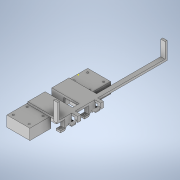
# Autodesk Inventor part: shell 6.0 screw
Saved by Autodesk Inventor 2020.2 (Build 242310000, 310)
## iProperties
Created: 2020-02-28
Part Number: shell 6.0 screw
Material: Generic
Document SubType Name: Modeling
Designer: ColinP
Density: 1 g/cm^3
Appearance: Default
Author: ColinP
Autodesk Inventor part; units mm, degrees
ref_plane "YZ Plane" through (0, 0, 0) normal (1, 0, 0) x (0, 1, 0)
ref_plane "XZ Plane" through (0, 0, 0) normal (0, 1, 0) x (-1, 0, 0)
ref_plane "XY Plane" through (0, 0, 0) normal (0, 0, 1) x (1, 0, 0)
sketch "Sketch1" plane through (0, 0, 0) normal (0, 1, 0) x (-1, 0, 0)
  line L0 (0, 0) -> (8, 0)
  line L1 (8, 0) -> (8, 98.298)
  line L2 (8, 98.298) -> (0, 98.298)
  line L3 (0, 98.298) -> (0, 0)
  line L4 (8, 0) -> (0, 0)
  line L5 (0, 0) -> (0, -4)
  line L6 (0, -4) -> (8, -4)
  line L7 (8, -4) -> (8, 0)
  line L8 (8, 98.298) -> (0, 98.298)
  line L9 (0, 98.298) -> (0, 102.298)
  line L10 (0, 102.298) -> (8, 102.298)
  line L11 (8, 102.298) -> (8, 98.298)
  dimension "d0" = 8
  dimension "d1" = 98.298
  dimension "d2" = 8
  dimension "d3" = 4
  dimension "d4" = 4
  constraints: 24 end point, 6 parallel, 3 horizontal, 3 perpendicular
  measures "d0" distance of L2.end L1.end
  measures "d1" distance of L1.end L0.end
  measures "d2" distance of L6.end L5.end
  measures "d3" distance of L5.end L4.end
  measures "d4" distance of L8.end L9.end
extrude "Extrusion1" add sketch "Sketch1" along normal blind 4 contours L3 L2 L1 L0
extrude "Extrusion2" add sketch "Sketch1" along normal blind 34 contours L0 L7 L6 L5
sketch "Sketch2" plane through (0, 0, 0) normal (0, -1, 0) x (1, 0, 0)
  line L0 (0, 0) -> (0, 19.558)
  line L1 (0, 98.298) -> (0, 0) projected
  line L2 (0, 19.558) -> (0, 35.6705)
  line L3 (0, 35.6705) -> (0, 48.3705)
  line L4 (0, 48.3705) -> (-8, 48.3705)
  line L5 (-8, 0) -> (-8, 98.298) projected
  line L6 (-8, 19.558) -> (-8, 48.3705)
  line L7 (0, 19.558) -> (-8, 19.558)
  dimension "d9" = 19.558
  dimension "d10" = 16.1125
  dimension "d11" = 12.7
  constraints: 12 end point, 5 point on line, 2 perpendicular, 1 collinear
  measures "d9" distance of L0.start L0.end
  measures "d10" distance of L0.end L2.end
  measures "d11" distance of L2.end L3.end
extrude "Extrusion3" add sketch "Sketch2" along normal blind 25
sketch "Sketch3" plane through (0, 0, -4) normal (1, 0, 0) x (0, 0, -1)
  line L0 (-52.3705, -25) -> (-23.558, -25)
  line L1 (-37.9642, -25) -> (-37.9642, -17.7991)
  line L2 (-37.9642, -17.7991) -> (-31.5508, -17.7991)
  line L3 (-31.5508, -17.7991) -> (-44.3778, -17.7991)
  line L4 (-44.3778, -17.7991) -> (-41.1646, -12.2338)
  line L5 (-44.3778, -17.7991) -> (-37.9516, -17.7991) construction
  line L6 (-41.1646, -12.2338) -> (-34.7385, -12.2338)
  line L7 (-34.7385, -12.2338) -> (-31.5253, -17.7991)
  line L8 (-31.5253, -17.7991) -> (-34.7385, -23.3644)
  line L9 (-34.7385, -23.3644) -> (-41.1647, -23.3644)
  line L10 (-41.1647, -23.3644) -> (-44.3778, -17.7991)
  line L11 (-23.558, 0) -> (-23.558, -25)
  line L12 (-52.3705, 0) -> (-52.3705, -25)
  line L13 (-23.558, -25) -> (-52.3705, -25)
  line L14 (-52.3705, -25) -> (-52.3705, -13.8875)
  line L15 (-23.558, -13.8875) -> (-23.558, -25)
  line L16 (-31.5253, -17.7991) -> (-23.558, -17.7991)
  line L17 (-44.3778, -17.7991) -> (-52.3705, -17.7991)
  point P0 (-4, 0)
  point P1 (-37.9642, -23.3644)
  dimension "d14" = 7.2009
  dimension "d15" = 6.4135
  dimension "d16" = 12.827
  dimension "d17" = 6.4262
  dimension "d18" = 60
  dimension "d19" = 6.4262
  dimension "d20" = 120
  dimension "d21" = 120
  dimension "d22" = 6.4262
  dimension "d23" = 120
  dimension "d24" = 6.4262
  dimension "d25" = 120
  constraints: 30 end point, 6 horizontal, 5 point on line, 3 parallel, 1 equal length, 1 midpoint, 1 perpendicular, 1 vertical
  measures "d14" distance of L1.start L1.end
  measures "d15" distance of L1.end L2.end
  measures "d16" distance of L2.end L3.end
  measures "d17" distance of L3.end L4.end
  measures "d18" angle of L5 L4
  measures "d19" distance of L4.end L6.end
  measures "d20" angle of L4 L6
  measures "d21" angle of L6 L7
  measures "d22" distance of L7.end L8.end
  measures "d23" angle of L7 L8
  measures "d24" distance of L8.end L9.end
  measures "d25" angle of L8 L9
extrude "Extrusion4" cut sketch "Sketch3" against normal blind 25.4
sketch "Sketch4" plane through (0, 0, -4) normal (1, 0, 0) x (0, 0, -1)
  line L0 (0, 0) -> (-23.558, 0) projected
  line L1 (-23.558, 0) -> (-29.558, 0)
  line L2 (-29.558, 0) -> (-29.558, -12.8016)
  line L3 (-29.558, -12.8016) -> (-23.558, -12.8016)
  line L4 (-23.558, -12.8016) -> (-23.558, 0)
  line L5 (-52.3705, 0) -> (-52.3705, -25) projected
  line L6 (-52.3705, 0) -> (-46.3761, 0)
  line L7 (-46.3761, 0) -> (-46.3761, -12.8016)
  line L8 (-46.3761, -12.8016) -> (-52.3705, -12.8016)
  line L9 (-52.3705, -12.8016) -> (-52.3705, 0)
  point P0 (-4, 0)
  point P1 (-52.3705, -13.8875)
  dimension "d28" = 6
  dimension "d29" = 12.8016
  dimension "d30" = 5.9944
  dimension "d31" = 12.8016
  constraints: 16 end point, 4 parallel, 2 horizontal, 2 perpendicular
  measures "d28" distance of L3.end L2.end
  measures "d29" distance of L2.end L1.end
  measures "d30" distance of L7.end L8.end
  measures "d31" distance of L6.end L7.end
extrude "Extrusion5" cut sketch "Sketch4" against normal blind 25.4
sketch "Sketch6" plane through (0, 0, -4) normal (1, 0, 0) x (0, 0, -1)
  line L0 (-29.558, -12.8016) -> (-29.558, 0) projected
  line L1 (-29.558, 0) -> (-31.558, 0)
  line L2 (-31.558, 0) -> (-31.558, -12.8016)
  line L3 (-31.558, -12.8016) -> (-29.558, -12.8016)
  line L4 (-29.558, -12.8016) -> (-29.558, 0)
  line L5 (-46.3761, -12.8016) -> (-46.3761, 0) projected
  line L6 (-46.3761, 0) -> (-44.3761, 0)
  line L7 (-44.3761, 0) -> (-44.3761, -12.8016)
  line L8 (-44.3761, -12.8016) -> (-46.3761, -12.8016)
  line L9 (-46.3761, -12.8016) -> (-46.3761, 0)
  point P0 (-4, 0)
  dimension "d44" = 2
  dimension "d45" = 12.8016
  dimension "d46" = 2
  constraints: 16 end point, 4 parallel, 2 horizontal, 2 perpendicular, 1 point on line
  measures "d44" distance of L3.end L2.end
  measures "d45" distance of L2.end L1.end
  measures "d46" distance of L7.end L8.end
extrude "Extrusion6" cut sketch "Sketch6" against normal blind 25.4
sketch "Sketch5" plane through (0, -17.7991, 19.558) normal (0, -1, 0) x (1, 0, 0)
  line L0 (-8, 0) -> (0, 0) projected
  line L1 (-4, 0) -> (-4, 28.8125)
  line L2 (-8, 28.8125) -> (0, 28.8125) projected
  line L3 (-4, 14.4063) -> (-4, 4.4063)
  line L4 (-4, 14.4063) -> (6, 14.4063) construction
  line L5 (-4, 4.4063) -> (-4, 24.4062)
  point P0 (0, -19.558)
  dimension "d34" = 10
  dimension "d35" = 90
  dimension "d36" = 20
  constraints: 8 end point, 3 midpoint, 1 horizontal, 1 perpendicular, 1 point on line, 1 vertical
  measures "d34" distance of L3.start L3.end
  measures "d35" angle of L3 L4
  measures "d36" distance of L3.end L5.end
hole "Hole1" at (-4, -17.7991, 23.9642) at (-4, -17.7991, 43.9642) direction (0, 1, 0) diameter 3.4 depth 4.9975 clearance for "Flat Head Machine Screw" size "M3" standard "Ansi Metric M Profile"
sketch "Sketch14" plane through (0, 4, 0) normal (0, 1, 0) x (1, 0, 0)
  line L0 (-8, -30.7385) -> (-8, -37.1647) projected
  line L1 (0, -30.7385) -> (-8, -30.7385) projected
  line L2 (0, -37.1647) -> (0, -30.7385) projected
  line L3 (0, -37.1647) -> (-8, -37.1647) projected
  line L4 (-8, -33.9515) -> (-8, -17.7115)
  line L5 (-8, -17.7115) -> (-59.53, -17.7116)
  line L6 (-59.53, -17.7116) -> (-59.53, -50.1916)
  line L7 (-59.53, -50.1916) -> (-8, -50.1915)
  line L8 (-8, -50.1915) -> (-8, -17.7115)
  point P0 (0, 0)
  point P1 (-8, -37.1647)
  point P2 (-8, -30.7385)
  dimension "d78" = 16.24
  dimension "d79" = 51.53
  dimension "d80" = 32.48
  dimension "d81" = 90
  dimension "d82" = 90
  constraints: 10 end point, 2 perpendicular, 1 midpoint
  measures "d78" distance of L4.start L4.end
  measures "d79" distance of L4.end L5.end
  measures "d80" distance of L5.end L6.end
  measures "d81" angle of L6 L5
  measures "d82" angle of L7 L6
extrude "Extrusion11" add sketch "Sketch14" against normal blind 4 contours L0 L8 L7 L6 L5 L4
sketch "Sketch15" plane through (0, 0, 0) normal (0, -1, 0) x (1, 0, 0)
  line L0 (-59.53, 19.7116) -> (-59.53, 17.7116)
  line L1 (-8, 17.7115) -> (-59.53, 17.7116) projected
  line L2 (-59.53, 17.7116) -> (-57.53, 17.7116)
  line L3 (-57.53, 17.7116) -> (-57.53, 19.7116)
  line L4 (-57.53, 19.7116) -> (-59.53, 19.7116)
  line L5 (-59.53, 19.7116) -> (-59.53, 17.7116)
  line L6 (-59.53, 50.1916) -> (-59.53, 17.7116) projected
  line L7 (-59.53, 50.1916) -> (-38.53, 50.1916)
  line L8 (-38.53, 50.1916) -> (-38.53, 48.1916)
  line L9 (-38.53, 48.1916) -> (-59.53, 48.1916)
  line L10 (-59.53, 48.1916) -> (-59.53, 50.1916)
  line L11 (-38.53, 48.1916) -> (-57.53, 48.1916)
  line L12 (-57.53, 48.1916) -> (-57.53, 19.7116)
  line L13 (-57.53, 19.7116) -> (-38.53, 19.7116)
  line L14 (-38.53, 19.7116) -> (-38.53, 48.1916)
  line L15 (-38.53, 19.7116) -> (-57.53, 19.7116)
  line L16 (-57.53, 19.7116) -> (-57.53, 17.7116)
  line L17 (-57.53, 17.7116) -> (-38.53, 17.7116)
  line L18 (-38.53, 17.7116) -> (-38.53, 19.7116)
  line L19 (-8, -4) -> (-8, 17.7115) projected
  line L20 (0, -4) -> (-8, -4) projected
  line L21 (0, 27.558) -> (0, -4) projected
  line L22 (0, 27.558) -> (-8, 27.558) projected
  line L23 (-8, 40.3761) -> (-8, 27.558) projected
  line L24 (0, 40.3761) -> (-8, 40.3761) projected
  line L25 (0, 98.298) -> (0, 40.3761) projected
  line L26 (-8, 50.1915) -> (-8, 98.298) projected
  line L27 (-8, 50.1915) -> (-59.53, 50.1916) projected
  line L28 (-59.53, 50.1916) -> (-59.53, 17.7116) projected
  line L29 (-59.53, 17.7116) -> (-8, 17.7115) projected
  line L30 (-8, 98.298) -> (0, 98.298) projected
  point P0 (0, 0)
  point P1 (-38.53, 17.7116)
  dimension "d87" = 2
  dimension "d88" = 2
  dimension "d89" = 21
  dimension "d90" = 2
  constraints: 34 end point, 8 parallel, 4 horizontal, 4 perpendicular
  measures "d87" distance of L4.end L3.end
  measures "d88" distance of L3.end L2.end
  measures "d89" distance of L8.end L9.end
  measures "d90" distance of L7.end L8.end
extrude "Extrusion12" add sketch "Sketch15" along normal blind 36 contours L4 L3 L1 L0 | L6 L9 L12 L4 | L13 L18 L1 L3 | L6 L7 L8 L9
sketch "Sketch16" plane through (-38.53, 0, 48.1916) normal (1, 0, 0) x (0, 0, -1)
  line L0 (7.8155, 0) -> (20.6335, 0) projected
  line L1 (14.2245, 0) -> (14.2245, -17.78)
  line L2 (14.2245, -17.78) -> (14.2245, -25.78)
  line L3 (14.2245, -25.78) -> (31.7245, -25.78)
  line L4 (31.7245, -25.78) -> (-3.2755, -25.78)
  line L5 (-3.2755, -25.78) -> (-3.2755, -22.28)
  line L6 (-3.2755, -22.28) -> (-2, -22.28)
  line L7 (-2, 0) -> (-2, -36) projected
  line L8 (-2, -22.28) -> (-7, -22.28)
  line L9 (-7, -22.28) -> (-7, -29.28)
  line L10 (-7, -22.28) -> (0, -22.28) construction
  line L11 (-7, -29.28) -> (-2, -29.28)
  line L12 (-2, -22.28) -> (-2, -29.28)
  line L13 (30.48, 0) -> (30.48, -36) projected
  line L14 (30.48, -29.28) -> (35.48, -29.28)
  line L15 (35.48, -29.28) -> (35.48, -22.28)
  line L16 (35.48, -22.28) -> (30.48, -22.28)
  circle A0 centre (-3.2755, -25.78) radius 1.7
  circle A1 centre (31.7245, -25.78) radius 1.7
  point P0 (48.1916, 0)
  point P1 (-2, -26.9039)
  point P2 (-3.2755, -24.08)
  point P3 (30.48, -24.6219)
  point P4 (30.48, -26.9381)
  point P5 (-2, -24.6561)
  point P6 (32.98, -22.28)
  point P7 (-3.5, -22.28)
  dimension "d93" = 17.78
  dimension "d94" = 8
  dimension "d95" = 180
  dimension "d96" = 17.5
  dimension "d97" = 90
  dimension "d98" = 35
  dimension "d99" = 3.5
  dimension "d100" = 5
  dimension "d101" = 7
  dimension "d102" = 90
  dimension "d103" = 5
  dimension "d104" = 3.4
  dimension "d105" = 3.4
  constraints: 28 end point, 8 perpendicular, 8 point on line, 3 midpoint, 2 centre point, 2 coincident, 2 vertical, 1 collinear, 1 horizontal, 1 horizontal alignment
  measures "d93" distance of L1.start L1.end
  measures "d94" distance of L1.end L2.end
  measures "d95" angle of L2 L1
  measures "d96" distance of L2.end L3.end
  measures "d97" angle of L3 L2
  measures "d98" distance of L3.end L4.end
  measures "d99" distance of L4.end L5.end
  measures "d100" distance of L6.end L8.end
  measures "d101" distance of L8.end L9.end
  measures "d102" angle of L9 L10
  measures "d103" distance of L14.start L14.end
  measures "d104" diameter of A0
  measures "d105" diameter of A1
extrude "Extrusion13" cut sketch "Sketch16" against normal blind 25.4 contours A1 L13 L3 | L3 L13 A1 | L13 A1 | A0 L7 L4 | L4 L7 A0 | L7 A0 L5 L4 | L4 L5 A0 L7
extrude "Extrusion14" add sketch "Sketch16" against normal blind 6.4262 contours L13 L16 L15 L14 A1 | A0 L5 L6 L7 | L7 L11 L9 L8 L5 A0
sketch "Sketch17" plane through (-59.53, 4, 17.7116) normal (-1, 0, 0) x (0, 0, 1)
  point P0 (-17.7115, -4)
sketch "Sketch18" plane through (-59.53, 4, 17.7116) normal (-1, 0, 0) x (0, 0, 1)
  line L0 (-5, -33.28) -> (0, -33.28) projected
  line L1 (0, -26.28) -> (-5, -26.28) projected
  line L2 (0, -33.28) -> (1.5, -33.28)
  line L3 (1.5, -33.28) -> (1.5, -26.28)
  line L4 (1.5, -26.28) -> (0, -26.28)
  line L5 (0, -26.28) -> (0, -33.28)
  line L6 (32.48, 0) -> (32.48, -40) projected
  line L7 (32.48, -26.28) -> (30.98, -26.28)
  line L8 (30.98, -26.28) -> (30.98, -33.28)
  line L9 (30.98, -33.28) -> (32.48, -33.28)
  line L10 (32.48, -33.28) -> (32.48, -26.28)
  point P0 (-17.7115, -4)
  point P1 (0.75, -33.28)
  point P2 (31.73, -33.28)
  dimension "d110" = 1.5
  dimension "d111" = 1.5
  constraints: 16 end point, 4 parallel, 2 horizontal, 2 midpoint, 2 perpendicular, 1 horizontal alignment, 1 point on line
  measures "d110" distance of L4.end L3.end
  measures "d111" distance of L9.end L8.end
extrude "Extrusion15" cut sketch "Sketch18" against normal up to surface (14.5738 mm away)
sketch "Sketch21" plane through (0, 0, 0) normal (0, -1, 0) x (1, 0, 0)
  line L0 (-8, 48.3705) -> (-8, 40.3761) projected
  line L1 (-8, 48.3705) -> (-8, 93.1705)
  line L2 (-8, 50.1915) -> (-8, 17.7115) projected
  line L3 (0, 98.298) -> (0, 0) projected
  line L4 (-8, 93.1705) -> (0, 93.1705)
  line L5 (0, 93.1705) -> (0, 64.3669)
  line L6 (0, 64.3669) -> (-8, 64.3669)
  line L7 (-8, 64.3669) -> (-8, 93.1705)
  point P0 (-8, 98.298)
  dimension "d128" = 44.8
  dimension "d129" = 28.8036
  constraints: 10 end point, 2 parallel, 2 point on line, 1 horizontal, 1 perpendicular
  measures "d128" distance of L0.start L1.end
  measures "d129" distance of L4.end L5.end
extrude "Extrusion18" add sketch "Sketch21" along normal blind 25.4
sketch "Sketch22" plane through (0, 0, -4) normal (1, 0, 0) x (0, 0, -1)
  line L0 (-68.3669, -25.4) -> (-97.1705, -25.4) projected
  line L1 (-82.7687, -25.4) -> (-82.7687, 0)
  line L2 (-82.7687, 0) -> (-82.7687, -12.2147)
  line L3 (-52.3705, -12.8016) -> (-44.3761, -12.8016) projected
  line L4 (-82.7687, -12.2147) -> (-85.9818, -12.2147)
  line L5 (-85.9818, -12.2147) -> (-89.1949, -17.78)
  line L6 (-82.7687, -12.2147) -> (-79.5556, -12.2147)
  line L7 (-79.5556, -12.2147) -> (-76.3425, -17.78)
  line L8 (-76.3425, -17.78) -> (-68.3669, -17.78)
  line L9 (-68.3669, -17.78) -> (-97.1705, -17.78)
  line L10 (-97.1705, 0) -> (-97.1705, -25.4) projected
  line L11 (-97.1705, -17.78) -> (-97.1705, 0)
  line L12 (-97.1705, 0) -> (-68.3669, 0)
  line L13 (-68.3669, 0) -> (-68.3669, -17.78)
  line L14 (-68.3669, -25.4) -> (-68.3669, -17.78)
  point P0 (-4, 0)
  point P1 (-89.1949, -17.78)
  dimension "d132" = 3.2131
  dimension "d133" = 6.4262
  dimension "d134" = 120
  dimension "d135" = 3.2131
  dimension "d136" = 6.4262
  dimension "d137" = 120
  dimension "d141" = 17.78
  constraints: 24 end point, 4 perpendicular, 2 horizontal, 2 point on line, 2 vertical, 1 midpoint, 1 parallel
  measures "d132" distance of L2.end L4.end
  measures "d133" distance of L4.end L5.end
  measures "d134" angle of L5 L4
  measures "d135" distance of L2.end L6.end
  measures "d136" distance of L6.end L7.end
  measures "d137" angle of L6 L7
  measures "d141" distance of L9.end L10.start
extrude "Extrusion19" cut sketch "Sketch22" against normal blind 25.4 contours L0 L1 L9 L8 L14 | L0 L10 L9 L1 | L9 L5 L4 L1 | L1 L6 L7 L9
sketch "Sketch23" plane through (0, 0, -4) normal (1, 0, 0) x (0, 0, -1)
  line L0 (-44.3761, -12.8016) -> (-52.3705, -12.8016) projected
  line L1 (-52.3705, -12.8016) -> (-68.3669, -12.8016)
  line L2 (-68.3669, 0) -> (-68.3669, -17.78) projected
  line L3 (-68.3669, -12.8016) -> (-76.3679, -12.8016)
  line L4 (-76.3679, -12.8016) -> (-76.3679, 0)
  line L5 (-54.1915, 0) -> (-68.3669, 0) projected
  line L6 (-76.3679, 0) -> (-68.3669, 0)
  line L7 (-68.3669, 0) -> (-68.3669, -12.8016)
  line L8 (-97.1705, 0) -> (-97.1705, -17.78) projected
  line L9 (-97.1705, -12.8016) -> (-89.1695, -12.8016)
  line L10 (-97.1705, -12.8016) -> (-89.1695, -12.8016) construction
  line L11 (-89.1695, -12.8016) -> (-89.1695, 0)
  line L12 (-89.1695, 0) -> (-97.1705, 0)
  line L13 (-97.1705, 0) -> (-97.1705, -12.8016)
  point P0 (-4, 0)
  point P1 (-72.3674, -12.8016)
  point P2 (-93.17, -12.8016)
  dimension "d140" = 8.001
  dimension "d142" = 8.001
  dimension "d143" = 0
  constraints: 20 end point, 6 perpendicular, 4 horizontal, 2 midpoint, 2 point on line, 1 collinear, 1 horizontal alignment
  measures "d140" distance of L1.end L3.end
  measures "d142" distance of L9.start L9.end
  measures "d143" distance between parallel lines of L9 L10
extrude "Extrusion20" cut sketch "Sketch23" against normal blind 25.4
sketch "Sketch24" plane through (0, -17.78, 85.1949) normal (0, -1, 0) x (1, 0, 0)
  line L0 (0, -3.2131) -> (-8, -3.2131) projected
  line L1 (0, -9.6393) -> (-8, -9.6393) projected
  line L2 (0, -3.2131) -> (0, -9.6393)
  line L3 (0, -6.4262) -> (-4, -6.4262)
  line L4 (-4, -6.4262) -> (-4, -16.4262)
  line L5 (-4, -16.4262) -> (-4, 3.5738)
  point P0 (0, -85.1949)
  dimension "d146" = 10
  dimension "d147" = 20
  constraints: 8 end point, 1 horizontal, 1 midpoint, 1 perpendicular, 1 point on line, 1 vertical
  measures "d146" distance of L3.end L4.end
  measures "d147" distance of L4.end L5.end
hole "Hole2" at (-4, -17.78, 68.7687) at (-4, -17.78, 88.7687) direction (0, 1, 0) diameter 3.4 depth 4.9784 clearance for "Flat Head Machine Screw" size "M3" standard "Ansi Metric M Profile"
sketch "Sketch25" plane through (0, 4, 0) normal (0, 1, 0) x (1, 0, 0)
  line L0 (-8, -75.5556) -> (-8, -81.9818) projected
  line L1 (0, -75.5556) -> (-8, -75.5556) projected
  line L2 (0, -81.9818) -> (0, -75.5556) projected
  line L3 (0, -81.9818) -> (-8, -81.9818) projected
  line L4 (-8, -50.1915) -> (-8, -17.7115) projected
  line L5 (-8, -78.7687) -> (-8, -62.5254)
  line L6 (-8, -62.5254) -> (-8, -95.012)
  line L7 (-8, -95.012) -> (0, -95.012)
  line L8 (0, -95.012) -> (0, -62.5254)
  line L9 (0, -98.298) -> (0, 0) projected
  line L10 (-8, -62.5254) -> (0, -62.5254)
  line L11 (-8, -62.5254) -> (-59.5366, -62.5254)
  line L12 (-59.5366, -62.5254) -> (-59.5366, -95.012)
  line L13 (-59.5366, -95.012) -> (-8, -95.012)
  point P0 (-8, -98.298)
  dimension "d155" = 16.2433
  dimension "d156" = 32.4866
  dimension "d157" = 51.5366
  constraints: 16 end point, 4 perpendicular, 4 point on line, 1 horizontal
  measures "d155" distance of L5.start L5.end
  measures "d156" distance of L5.end L6.end
  measures "d157" distance of L5.end L11.end
extrude "Extrusion21" add sketch "Sketch25" against normal blind 4 contours L0 L6 L13 L12 L11 L5
sketch "Sketch26" plane through (0, 0, 0) normal (0, -1, 0) x (1, 0, 0)
  line L0 (-59.5366, 95.012) -> (-59.5366, 62.5254) projected
  line L1 (-8, 95.012) -> (-59.5366, 95.012) projected
  line L2 (-59.5366, 62.5254) -> (-38.5366, 62.5254)
  line L3 (-38.5366, 62.5254) -> (-38.5366, 95.012)
  line L4 (-38.5366, 95.012) -> (-59.5366, 95.012)
  line L5 (-59.5366, 95.012) -> (-59.5366, 62.5254)
  line L6 (-38.5366, 62.5254) -> (-40.5366, 62.5254)
  line L7 (-40.5366, 62.5254) -> (-40.5366, 64.5254)
  line L8 (-40.5366, 64.5254) -> (-38.5366, 64.5254)
  line L9 (-38.5366, 64.5254) -> (-38.5366, 62.5254)
  line L10 (-59.5366, 95.012) -> (-57.5366, 95.012)
  line L11 (-57.5366, 95.012) -> (-57.5366, 93.012)
  line L12 (-57.5366, 93.012) -> (-59.5366, 93.012)
  line L13 (-59.5366, 93.012) -> (-59.5366, 95.012)
  line L14 (-57.5366, 93.012) -> (-40.5366, 93.012)
  line L15 (-40.5366, 93.012) -> (-40.5366, 64.5254)
  line L16 (-40.5366, 64.5254) -> (-57.5366, 64.5254)
  line L17 (-57.5366, 64.5254) -> (-57.5366, 93.012)
  line L18 (-40.5366, 93.012) -> (-40.5366, 95.012)
  point P0 (0, 0)
  point P1 (-40.5366, 62.5254)
  dimension "d160" = 21
  dimension "d161" = 2
  dimension "d162" = 2
  dimension "d163" = 2
  dimension "d164" = 2
  constraints: 34 end point, 8 parallel, 5 perpendicular, 4 horizontal, 2 point on line
  measures "d160" distance of L4.end L3.end
  measures "d161" distance of L7.end L8.end
  measures "d162" distance of L6.end L7.end
  measures "d163" distance of L11.end L12.end
  measures "d164" distance of L10.end L11.end
extrude "Extrusion22" add sketch "Sketch26" along normal blind 36 contours L1 L11 L12 L0 | L12 L17 L16 L7 L2 L0 | L1 L18 L14 L11
sketch "Sketch27" plane through (-40.5366, 0, 95.012) normal (1, 0, 0) x (0, 0, -1)
  line L0 (39.8204, -22.28) -> (39.8204, -29.28) projected
  line L1 (39.8204, -22.28) -> (32.4866, -22.28)
  line L2 (32.4866, 4) -> (32.4866, -36) projected
  line L3 (32.4866, -22.28) -> (32.4866, -29.28)
  line L4 (32.4866, -29.28) -> (37.4866, -29.28)
  line L5 (37.4866, -29.28) -> (37.4866, -22.28)
  line L6 (0, 4) -> (0, -36) projected
  line L7 (0, -29.28) -> (-5, -29.28)
  line L8 (-5, -29.28) -> (-5, -22.28)
  line L9 (-5, -22.28) -> (0, -22.28)
  circle A0 centre (43.545, -25.78) radius 1.7 projected
  line L10 (43.545, -25.78) -> (16.2433, -25.78)
  line L11 (19.4564, -12.2147) -> (13.0302, -12.2147) projected
  line L12 (16.2433, -25.78) -> (33.7433, -25.78)
  line L13 (33.7433, -25.78) -> (-1.2567, -25.78)
  circle A1 centre (-1.2567, -25.78) radius 1.7
  circle A2 centre (33.7433, -25.78) radius 1.7
  point P0 (95.012, 0)
  point P1 (0, -26.9249)
  point P2 (0, -24.6351)
  point P3 (32.4866, -24.6351)
  point P4 (32.4866, -26.9249)
  point P5 (32.4866, 0)
  point P6 (0, 0)
  dimension "d167" = 7
  dimension "d168" = 5
  dimension "d169" = 5
  dimension "d170" = 17.5
  dimension "d171" = 35
  dimension "d172" = 3.4
  dimension "d173" = 3.4
  constraints: 20 end point, 10 point on line, 3 perpendicular, 2 centre point, 2 coincident, 1 horizontal, 1 parallel, 1 vertical
  measures "d167" distance of L1.end L3.end
  measures "d168" distance of L3.end L4.end
  measures "d169" distance of L7.start L7.end
  measures "d170" distance of L10.end L12.end
  measures "d171" distance of L12.end L13.end
  measures "d172" diameter of A1
  measures "d173" diameter of A2
extrude "Extrusion23" add sketch "Sketch27" against normal blind 5 contours L5 L10 A2 L2 L1 | L5 L4 L2 A2 L10 | L6 A1 L7 L8 L9
extrude "Extrusion24" cut sketch "Sketch27" against normal up to surface (19 mm away) contours L2 L10 A2 | A2 L10 L2 | A1 L13 L6 | L13 A1 L6 picked at (32.4062, -25.1304) picked at (32.4062, -26.4296)
sketch "Sketch28" plane through (-59.5366, 4, 62.5254) normal (-1, 0, 0) x (0, 0, 1)
  line L0 (0, -33.28) -> (-5, -33.28) projected
  line L1 (0, -33.28) -> (1.5, -33.28)
  line L2 (1.5, -33.28) -> (1.5, -26.28)
  line L3 (1.5, -26.28) -> (0, -26.28)
  line L4 (0, -26.28) -> (0, -33.28)
  line L5 (37.4866, -33.28) -> (32.4866, -33.28) projected
  line L6 (32.4866, -33.28) -> (30.9866, -33.28)
  line L7 (30.9866, -33.28) -> (30.9866, -26.28)
  line L8 (30.9866, -26.28) -> (32.4866, -26.28)
  line L9 (32.4866, -26.28) -> (32.4866, -33.28)
  point P0 (-62.5254, -4)
  dimension "d178" = 1.5
  dimension "d179" = 1.5
  constraints: 16 end point, 4 parallel, 2 horizontal, 2 perpendicular, 1 point on line
  measures "d178" distance of L3.end L2.end
  measures "d179" distance of L7.end L8.end
extrude "Extrusion25" cut sketch "Sketch28" against normal up to surface (14 mm away)
sketch "Sketch29" plane through (0, 4, 0) normal (0, 1, 0) x (1, 0, 0)
  line L0 (-8, -17.7115) -> (-59.53, -17.7116) projected
  line L1 (-8, -17.7115) -> (11.05, -17.7115)
  line L2 (11.05, -17.7115) -> (11.05, -7.7115)
  line L3 (11.05, -7.7115) -> (-8, -7.7116)
  line L4 (-8, -7.7116) -> (-8, -17.7115)
  line L5 (11.05, -17.7115) -> (5.97, -17.7115)
  line L6 (5.97, -17.7115) -> (5.97, -7.7115)
  line L7 (5.97, -7.7115) -> (11.05, -7.7115)
  line L8 (11.05, -7.7115) -> (11.05, -17.7115)
  point P0 (0, 0)
  dimension "d182" = 19.05
  dimension "d183" = 10
  dimension "d184" = 5.08
  constraints: 16 end point, 4 parallel, 2 horizontal, 2 perpendicular, 1 point on line
  measures "d182" distance of L3.end L2.end
  measures "d183" distance of L2.end L1.end
  measures "d184" distance of L6.end L7.end
extrude "Extrusion26" add sketch "Sketch29" against normal blind 4 contours L4 L3 L6 L1
extrude "Extrusion27" add sketch "Sketch29" against normal blind 10 contours L6 L3 L2 L1
sketch "Sketch30" plane through (0, 0, 17.7115) normal (0, 0, 1) x (1, 0, 0)
  line L0 (11.05, -6) -> (5.97, -6) projected
  line L1 (8.51, -6) -> (8.51, -4)
  circle A0 centre (8.51, -4) radius 1.5
  point P0 (0, 0)
  dimension "d189" = 2
  dimension "d190" = 3
  constraints: 2 end point, 1 centre point, 1 coincident, 1 midpoint, 1 vertical
  measures "d189" distance of L1.start L1.end
  measures "d190" diameter of A0
extrude "Extrusion28" add sketch "Sketch30" along normal blind 25.4
sketch "Sketch32" plane through (0, 34, 0) normal (0, 1, 0) x (1, 0, 0)
  line L0 (0, 4) -> (-8, 4) projected
  line L1 (-8, 4) -> (-8, 0) projected
  line L2 (-8, 0) -> (0, 0) projected
  line L3 (0, 0) -> (0, 4) projected
extrude "Extrusion29" cut sketch "Sketch32" against normal blind 30
sketch "Sketch33" plane through (0, 0, -4) normal (0, 0, -1) x (-1, 0, 0)
  line L0 (8, 4) -> (0, 4) projected
  line L1 (0, 0) -> (0, 4) projected
  line L2 (0, 0) -> (8, 0) projected
  line L3 (8, 0) -> (8, 4) projected
  point P0 (0, 0)
extrude "Extrusion30" add sketch "Sketch33" along normal blind 102.489
sketch "Sketch35" plane through (0, 0, 17.7115) normal (0, 0, 1) x (1, 0, 0)
  line L0 (0, 4) -> (11.05, 4) projected
  circle A0 centre (8.51, -4) radius 1.5 projected
  line L1 (0, 0) -> (0, 4) projected
  line L2 (5.97, 0) -> (0, 0) projected
  line L3 (5.97, 0) -> (5.97, -6) projected
  line L4 (11.05, -6) -> (5.97, -6) projected
  line L5 (11.05, 4) -> (11.05, -6) projected
  line L6 (0, 4) -> (11.05, 4) projected
  point P0 (0, 0)
extrude "Extrusion32" add sketch "Sketch35" along normal blind 11.43 contours L0 L5 L4 L3 L2 L1 | A0
sketch "Sketch42" plane through (11.05, -6, 7.7115) normal (1, 0, 0) x (0, 0, -1)
  line L0 (-21.43, 10) -> (0, 10) projected
  line L1 (0, 0) -> (-15.7974, 0)
  line L2 (-15.7974, 0) -> (-15.7974, 10)
  line L3 (-15.7974, 10) -> (0, 10)
  line L4 (0, 10) -> (0, 0)
  point P0 (7.7115, 6)
  point P1 (0, 10)
  constraints: 8 end point, 2 parallel, 1 horizontal, 1 perpendicular, 1 point on line
extrude "Extrusion38" cut sketch "Sketch42" against normal up to surface (11.05 mm away)
sketch "Sketch43" plane through (0, -12.8016, 93.1705) normal (0, 1, 0) x (1, 0, 0)
  circle A0 centre (-4, 4.4018) radius 1.7 projected
  line L0 (-8, 0) -> (-8, 8.001) projected
  line L1 (0, 0) -> (-8, 0) projected
  line L2 (0, 8.001) -> (0, 0) projected
  line L3 (0, 8.001) -> (-8, 8.001) projected
  circle A1 centre (-4, 24.4018) radius 1.7 projected
  line L4 (-8, 20.8026) -> (-8, 28.8036) projected
  line L5 (0, 20.8026) -> (-8, 20.8026) projected
  line L6 (0, 28.8036) -> (0, 20.8026) projected
  line L7 (-8, 28.8036) -> (0, 28.8036) projected
  line L8 (-8, 44.8) -> (-8, 52.7944) projected
  line L9 (0, 44.8) -> (-8, 44.8) projected
  line L10 (0, 52.7944) -> (0, 44.8) projected
  line L11 (-8, 65.6125) -> (-8, 73.6125) projected
  line L12 (0, 73.6125) -> (0, 65.6125) projected
  line L13 (-8, 73.6125) -> (0, 73.6125) projected
  circle A2 centre (-4, 49.2063) radius 1.7 projected
  circle A3 centre (-4, 69.2062) radius 1.7 projected
  line L14 (0, 65.6125) -> (-8, 65.6125) projected
  line L15 (0, 52.7944) -> (-8, 52.7944) projected
  point P0 (0, 93.1705)
extrude "Extrusion39" cut sketch "Sketch43" against normal blind 1.5 contours L0 L3 L2 L1 | A1 | L4 L7 L6 L5 | L8 L15 L10 L9 | L11 L13 L12 L14
sketch "Sketch44" plane through (0, 0, 0) normal (0, 1, 0) x (1, 0, 0)
  line L0 (-59.5366, -95.012) -> (-20.5366, -95.012)
  line L1 (-20.5366, -95.012) -> (-20.5366, -130.012)
  line L2 (-20.5366, -130.012) -> (-59.5366, -130.012)
  line L3 (-59.5366, -130.012) -> (-59.5366, -95.012)
  line L4 (-59.53, -50.1916) -> (-59.53, -17.7116) projected
  line L5 (-59.53, -17.7116) -> (-20.53, -17.7116)
  line L6 (-20.53, -17.7116) -> (-20.53, 17.2884)
  line L7 (-20.53, 17.2884) -> (-59.53, 17.2884)
  line L8 (-59.53, 17.2884) -> (-59.53, -17.7116)
  point P0 (0, 0)
  dimension "d243" = 39
  dimension "d244" = 35
  dimension "d245" = 39
  dimension "d246" = 35
  constraints: 16 end point, 4 parallel, 2 horizontal, 2 perpendicular
  measures "d243" distance of L1.end L2.end
  measures "d244" distance of L0.end L1.end
  measures "d245" distance of L7.end L6.end
  measures "d246" distance of L6.end L5.end
extrude "Extrusion40" add sketch "Sketch44" against normal blind 3
sketch "Sketch45" plane through (0, 4, 0) normal (0, 1, 0) x (1, 0, 0)
  line L0 (-59.53, 17.2884) -> (-59.53, -50.1916) projected
  line L1 (-59.53, 17.2884) -> (-54.53, 17.2884)
  line L2 (-54.53, 17.2884) -> (-54.53, 12.2884)
  line L3 (-54.53, 12.2884) -> (-59.53, 12.2884)
  line L4 (-59.53, 12.2884) -> (-59.53, 17.2884)
  line L5 (-54.53, 12.2884) -> (-24.83, 12.2884)
  line L6 (-24.83, 12.2884) -> (-24.83, -13.7616)
  line L7 (-24.83, -13.7616) -> (-54.53, -13.7616)
  line L8 (-54.53, -13.7616) -> (-54.53, 12.2884)
  line L9 (-59.5366, -62.5254) -> (-59.5366, -130.012) projected
  line L10 (-59.5366, -130.012) -> (-55.5366, -130.012)
  line L11 (-55.5366, -130.012) -> (-55.5366, -126.012)
  line L12 (-55.5366, -126.012) -> (-59.5366, -126.012)
  line L13 (-59.5366, -126.012) -> (-59.5366, -130.012)
  line L14 (-55.5366, -126.012) -> (-25.8366, -126.012)
  line L15 (-25.8366, -126.012) -> (-25.8366, -99.962)
  line L16 (-25.8366, -99.962) -> (-55.5366, -99.962)
  line L17 (-55.5366, -99.962) -> (-55.5366, -126.012)
  point P0 (0, 0)
  point P1 (-59.5366, -95.012)
  dimension "d249" = 5
  dimension "d250" = 5
  dimension "d251" = 29.7
  dimension "d252" = 26.05
  dimension "d253" = 4
  dimension "d254" = 4
  dimension "d255" = 29.7
  dimension "d256" = 26.05
  constraints: 32 end point, 8 parallel, 4 horizontal, 4 perpendicular
  measures "d249" distance of L2.end L3.end
  measures "d250" distance of L1.end L2.end
  measures "d251" distance of L6.end L7.end
  measures "d252" distance of L5.end L6.end
  measures "d253" distance of L12.end L11.end
  measures "d254" distance of L11.end L10.end
  measures "d255" distance of L16.end L15.end
  measures "d256" distance of L15.end L14.end
hole "Hole4" at (-25.8366, 4, 99.962) at (-55.5366, 4, 99.962) at (-25.8366, 4, 126.012) at (-55.5366, 4, 126.012) at (-24.83, 4, 13.7616) at (-24.83, 4, -12.2884) at (-54.53, 4, -12.2884) at (-54.53, 4, 13.7616) direction (0, -1, 0) diameter 3.4 end through all clearance for "Flat Head Machine Screw" size "M3" standard "Ansi Metric M Profile"
sketch "Sketch48" plane through (0, 4, 0) normal (0, 1, 0) x (1, 0, 0)
  line L0 (0, -23.5089) -> (0, 106.489) projected
  line L1 (-8, -17.7115) -> (-8, 106.489) projected
  line L2 (0, 106.489) -> (-8, 106.489)
  line L3 (-8, 106.489) -> (-8, 102.489)
  line L4 (-8, 102.489) -> (0, 102.489)
  line L5 (0, 102.489) -> (0, 106.489)
  point P0 (0, 0)
  point P1 (-8, 106.489)
  point P2 (0, 102.489)
  dimension "d271" = 4
  constraints: 8 end point, 2 parallel, 1 horizontal, 1 perpendicular, 1 point on line
  measures "d271" distance of L3.end L2.end
extrude "Extrusion43" add sketch "Sketch48" along normal blind 28.4
sketch "Sketch49" plane through (-40.5366, 0, 95.012) normal (1, 0, 0) x (0, 0, -1)
  circle A0 centre (-1.2567, -25.78) radius 1.7 projected
  line L0 (0, -29.28) -> (0, -36) projected
  line L1 (2, -36) -> (0, -36) projected
  line L2 (2, 0) -> (2, -36) projected
  line L3 (0, 0) -> (2, 0) projected
  line L4 (0, 0) -> (0, -3) projected
  line L5 (0, -22.28) -> (-5, -22.28) projected
  line L6 (-5, -22.28) -> (-5, -29.28) projected
  line L7 (-5, -29.28) -> (0, -29.28) projected
  circle A1 centre (33.7433, -25.78) radius 1.7 projected
  line L8 (32.4866, 0) -> (32.4866, -22.28) projected
  line L9 (30.4866, 0) -> (32.4866, 0) projected
  line L10 (30.4866, 0) -> (30.4866, -36) projected
  line L11 (32.4866, -36) -> (30.4866, -36) projected
  line L12 (32.4866, -29.28) -> (32.4866, -36) projected
  line L13 (32.4866, -29.28) -> (37.4866, -29.28) projected
  line L14 (37.4866, -29.28) -> (37.4866, -22.28) projected
  line L15 (37.4866, -22.28) -> (32.4866, -22.28) projected
  line L16 (0, -3) -> (0, -22.28) projected
  point P0 (95.012, 0)
extrude "Extrusion44" add sketch "Sketch49" along normal up to surface (2.0066 mm away)
sketch "Sketch50" plane through (0, 4, 0) normal (0, 1, 0) x (1, 0, 0)
  line L0 (0, 102.489) -> (-8, 102.489) projected
  line L1 (-8, -17.7115) -> (-8, 102.489) projected
  line L2 (-8, -17.7115) -> (-59.53, -17.7116) projected
  line L3 (-59.53, -17.7116) -> (-59.53, -50.1916) projected
  line L4 (-59.53, -50.1916) -> (-8, -50.1915) projected
  line L5 (-8, -50.1915) -> (-8, -62.5254) projected
  line L6 (-8, -62.5254) -> (-59.5366, -62.5254) projected
  line L7 (-59.5366, -62.5254) -> (-59.5366, -95.012) projected
  line L8 (-59.5366, -95.012) -> (-8, -95.012) projected
  line L9 (-8, -95.012) -> (-8, -98.298) projected
  line L10 (-8, -98.298) -> (0, -98.298) projected
  line L11 (0, -98.298) -> (0, -29.1416) projected
  line L12 (11.05, -29.1416) -> (0, -29.1416) projected
  line L13 (11.05, -29.1416) -> (11.05, -23.5089) projected
  line L14 (11.05, -23.5089) -> (0, -23.5089) projected
  line L15 (0, -23.5089) -> (0, 102.489) projected
  line L16 (-8, -95.012) -> (-8, -98.298) projected
  line L17 (-8, -95.012) -> (-8, -98.298)
  line L18 (-8, -98.298) -> (0, -98.298) projected
  line L19 (-8, -98.298) -> (0, -98.298)
  line L20 (0, -98.298) -> (0, -94.869)
  line L21 (0, -98.298) -> (0, -85.1695) projected
  line L22 (0, -94.869) -> (-8, -94.869)
  line L23 (0, -94.869) -> (8, -94.869) construction
  line L24 (-8, -94.869) -> (-8, -98.298)
  point P0 (0, 0)
  dimension "d276" = 3.429
  dimension "d277" = 180
  constraints: 12 end point, 3 collinear, 2 point on line, 1 horizontal
  measures "d276" distance of L10.end L20.end
  measures "d277" angle of L22 L23
extrude "Extrusion45" add sketch "Sketch50" along normal blind 30 contours L11 L10 L9 L24 L22
sketch "Sketch51" plane through (0, -13.8875, 48.3705) normal (1, 0, 0) x (0, 0, -1)
  line L0 (-44.6415, 13.8875) -> (-16.1549, 13.8875) projected
  line L1 (-46.4985, 17.8875) -> (19.2289, 17.8875) projected
  line L2 (-23.9441, 13.8875) -> (-17.5941, 13.8875)
  line L3 (-17.5941, 13.8875) -> (-17.5941, 17.8875)
  line L4 (-17.5941, 17.8875) -> (-23.9441, 17.8875)
  line L5 (-23.9441, 17.8875) -> (-23.9441, 13.8875)
  point P0 (48.3705, 13.8875)
  point P1 (-17.5941, 13.8875)
  dimension "d280" = 6.35
  constraints: 8 end point, 2 parallel, 2 point on line, 1 horizontal, 1 perpendicular
  measures "d280" distance of L4.end L3.end
extrude "Extrusion46" add sketch "Sketch51" along normal up to surface (11.05 mm away)
sketch "Sketch52" plane through (0, 0, 0) normal (0, -1, 0) x (1, 0, 0)
  line L0 (0, 65.9646) -> (11.05, 65.9646) projected
  line L1 (0, 72.3146) -> (11.05, 72.3146) projected
  line L2 (11.05, 65.9646) -> (5.97, 65.9646)
  line L3 (5.97, 65.9646) -> (5.97, 72.3146)
  line L4 (5.97, 72.3146) -> (11.05, 72.3146)
  line L5 (11.05, 72.3146) -> (11.05, 65.9646)
  point P0 (0, 0)
  dimension "d283" = 5.08
  constraints: 8 end point, 2 parallel, 1 horizontal, 1 perpendicular, 1 point on line
  measures "d283" distance of L3.end L4.end
extrude "Extrusion47" add sketch "Sketch52" along normal up to surface (6 mm away)
sketch "Sketch53" plane through (-38.53, -36, 19.7116) normal (1, 0, 0) x (0, 0, -1)
  line L0 (2, 36) -> (2, 33) projected
  line L1 (0, 36) -> (2, 36) projected
  line L2 (0, 36) -> (0, 0) projected
  line L3 (2, 0) -> (0, 0) projected
  line L4 (2, 6.72) -> (2, 0) projected
  line L5 (2, 6.72) -> (7, 6.72) projected
  line L6 (7, 6.72) -> (7, 13.72) projected
  line L7 (7, 13.72) -> (2, 13.72) projected
  line L8 (2, 33) -> (2, 13.72) projected
  circle A0 centre (3.2445, 10.22) radius 1.7 projected
  line L9 (-30.48, 6.72) -> (-30.48, 0) projected
  line L10 (-28.48, 0) -> (-30.48, 0) projected
  line L11 (-28.48, 36) -> (-28.48, 0) projected
  line L12 (-30.48, 36) -> (-28.48, 36) projected
  line L13 (-30.48, 36) -> (-30.48, 13.72) projected
  line L14 (-30.48, 13.72) -> (-35.48, 13.72) projected
  line L15 (-35.48, 13.72) -> (-35.48, 6.72) projected
  line L16 (-35.48, 6.72) -> (-30.48, 6.72) projected
  circle A1 centre (-31.7555, 10.22) radius 1.7 projected
  line L17 (-44.8138, 36) -> (-42.8138, 36) projected
  line L18 (-44.8138, 0) -> (-44.8138, 36) projected
  line L19 (-42.8138, 0) -> (-44.8138, 0) projected
  line L20 (-42.8138, 6.72) -> (-42.8138, 0) projected
  line L21 (-37.8138, 6.72) -> (-42.8138, 6.72) projected
  line L22 (-37.8138, 13.72) -> (-37.8138, 6.72) projected
  line L23 (-42.8138, 13.72) -> (-37.8138, 13.72) projected
  line L24 (-42.8138, 36) -> (-42.8138, 13.72) projected
  circle A2 centre (-41.5571, 10.22) radius 1.7 projected
  circle A3 centre (-76.5571, 10.22) radius 1.7 projected
  line L25 (-75.3004, 36) -> (-73.3004, 36) projected
  line L26 (-75.3004, 33) -> (-75.3004, 36) projected
  line L27 (-75.3004, 13.72) -> (-75.3004, 33) projected
  line L28 (-80.3004, 13.72) -> (-75.3004, 13.72) projected
  line L29 (-80.3004, 6.72) -> (-80.3004, 13.72) projected
  line L30 (-75.3004, 6.72) -> (-80.3004, 6.72) projected
  line L31 (-75.3004, 0) -> (-75.3004, 6.72) projected
  line L32 (-73.3004, 0) -> (-75.3004, 0) projected
  line L33 (-73.3004, 36) -> (-73.3004, 0) projected
  point P0 (19.7116, 36)
extrude "Extrusion48" add sketch "Sketch53" along normal blind 2
sketch "Sketch54" plane through (0, 0, 72.3146) normal (0, 0, 1) x (1, 0, 0)
  circle A0 centre (8.51, -4) radius 1.5 projected
  circle A1 centre (8.51, -4) radius 1
  point P0 (0, 0)
  constraints: 1 centre point, 1 coincident
extrude "Extrusion49" add sketch "Sketch54" along normal blind 12.7 contours A0 | A1
sketch "Sketch55" plane through (0, 0, 0) normal (0, 1, 0) x (1, 0, 0)
  line L0 (-20.53, -17.7116) -> (-20.53, 17.2884) projected
  line L1 (-20.53, -17.7116) -> (-18.53, -17.7116)
  line L2 (-20.53, -17.7116) -> (-8, -17.7115) projected
  line L3 (-18.53, -17.7116) -> (-61.5256, -17.7116)
  line L4 (-61.5256, -17.7116) -> (-61.5256, 19.2896)
  line L5 (-61.5256, 19.2896) -> (-18.53, 19.2896)
  line L6 (-18.53, 19.2896) -> (-18.53, -17.7116)
  line L7 (-59.5366, -95.012) -> (-8, -95.012) projected
  line L8 (-18.53, -95.012) -> (-61.5256, -95.012)
  line L9 (-61.5256, -95.012) -> (-61.5256, -132.0132)
  line L10 (-61.5256, -132.0132) -> (-18.53, -132.0132)
  line L11 (-18.53, -132.0132) -> (-18.53, -95.012)
  circle A0 centre (-54.53, 12.2884) radius 1.7 projected
  circle A1 centre (-24.83, -13.7616) radius 1.7 projected
  circle A2 centre (-24.83, 12.2884) radius 1.7 projected
  circle A3 centre (-54.53, -13.7616) radius 1.7 projected
  line L12 (-20.53, -17.7116) -> (-36.53, -17.7116) projected
  line L13 (-36.53, -17.7116) -> (-59.53, -17.7116) projected
  line L14 (-59.53, -17.7116) -> (-59.53, 17.2884) projected
  line L15 (-59.53, 17.2884) -> (-20.53, 17.2884) projected
  line L16 (-20.53, 17.2884) -> (-20.53, -17.7116) projected
  circle A4 centre (-25.8366, -126.012) radius 1.7 projected
  circle A5 centre (-25.8366, -99.962) radius 1.7 projected
  circle A6 centre (-55.5366, -99.962) radius 1.7 projected
  circle A7 centre (-55.5366, -126.012) radius 1.7 projected
  line L17 (-20.5366, -95.012) -> (-20.5366, -130.012) projected
  line L18 (-20.5366, -130.012) -> (-59.5366, -130.012) projected
  line L19 (-59.5366, -130.012) -> (-59.5366, -95.012) projected
  line L20 (-59.5366, -95.012) -> (-36.53, -95.012) projected
  line L21 (-36.53, -95.012) -> (-20.5366, -95.012) projected
  line L22 (-59.5366, -95.012) -> (-59.5366, -62.5254) projected
  line L23 (-61.5256, -95.012) -> (-59.5366, -95.012)
  line L24 (-59.5366, -95.012) -> (-59.5366, -93.012)
  line L25 (-59.5366, -93.012) -> (-61.5256, -93.012)
  line L26 (-61.5256, -93.012) -> (-61.5256, -95.012)
  line L27 (-61.5256, -17.7116) -> (-59.5256, -17.7116)
  line L28 (-59.5256, -17.7116) -> (-59.5256, -20.1226)
  line L29 (-59.5256, -20.1226) -> (-61.5256, -20.1226)
  line L30 (-61.5256, -20.1226) -> (-61.5256, -17.7116)
  line L31 (-18.53, -17.7116) -> (-33.5386, -17.7116)
  line L32 (-33.5386, -17.7116) -> (-33.5386, -19.7116)
  line L33 (-33.5386, -19.7116) -> (-18.53, -19.7116)
  line L34 (-18.53, -19.7116) -> (-18.53, -17.7116)
  line L35 (-18.53, -95.012) -> (-33.5386, -95.012)
  line L36 (-33.5386, -95.012) -> (-33.5386, -93.012)
  line L37 (-33.5386, -93.012) -> (-18.53, -93.012)
  line L38 (-18.53, -93.012) -> (-18.53, -95.012)
  point P0 (0, 0)
  dimension "d290" = 2
  dimension "d291" = 42.9956
  dimension "d292" = 37.0012
  dimension "d293" = 37.0012
  dimension "d294" = 2
  dimension "d295" = 2
  dimension "d298" = 15.0086
  dimension "d299" = 2
  constraints: 50 end point, 12 parallel, 6 horizontal, 6 perpendicular, 4 point on line
  measures "d290" distance of L0.start L1.end
  measures "d291" distance of L4.end L5.end
  measures "d292" distance of L3.end L4.end
  measures "d293" distance of L9.end L8.end
  measures "d294" distance of L24.end L23.end
  measures "d295" distance of L28.end L29.end
  measures "d298" distance of L33.end L32.end
  measures "d299" distance of L32.end L31.end
extrude "Extrusion50" add sketch "Sketch55" against normal blind 20 contours L0 L15 L14 L3 L4 L5 L6 L1 | L1 L34 L33 L32 L3 | L3 L28 L29 L30 | L19 L18 L17 L7 L11 L10 L9 L8 | L8 L26 L25 L22 | L36 L37 L38 L7
body "Solid1"
